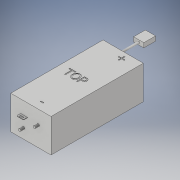
# Autodesk Inventor part: 12S Module
Saved by Autodesk Inventor 2017 (Build 210142000, 142)
## iProperties
Created: 2021-02-12
Part Number: 12S Module
Material: Generic
Document SubType Name: Modeling
Designer: Win240
Density: 1 g/cm^3
Appearance: Default
Author: Win240
Autodesk Inventor part; units mm, degrees
ref_plane "YZ Plane" through (0, 0, 0) normal (1, 0, 0) x (0, 1, 0)
ref_plane "XZ Plane" through (0, 0, 0) normal (0, 1, 0) x (-1, 0, 0)
ref_plane "XY Plane" through (0, 0, 0) normal (0, 0, 1) x (1, 0, 0)
sketch "Sketch1" plane through (0, 0, 0) normal (0, 0, 1) x (1, 0, 0)
  line L0 (-65.0875, -53.975) -> (65.0875, -53.975)
  line L1 (65.0875, -53.975) -> (65.0875, 53.975)
  line L2 (65.0875, 53.975) -> (-65.0875, 53.975)
  line L3 (-65.0875, 53.975) -> (-65.0875, -53.975)
  line L4 (-65.0875, -53.975) -> (65.0875, 53.975) construction
  line L5 (65.0875, -53.975) -> (-65.0875, 53.975) construction
  point P0 (0, 0)
  dimension "d0" = 130.175
  dimension "d1" = 107.95
  constraints: 12 end point, 2 midpoint, 2 parallel, 1 horizontal, 1 perpendicular
  measures "d0" distance of L0.start L0.end
  measures "d1" distance of L0.end L1.end
extrude "Extrusion1" add sketch "Sketch1" along normal blind 298.45
sketch "Sketch2" plane through (0, 0, 298.45) normal (0, 0, 1) x (1, 0, 0)
  line L0 (-65.0875, -53.975) -> (65.0875, -53.975) construction
  line L1 (-65.0875, 53.975) -> (-65.0875, -53.975) construction
  circle A0 centre (-23.8125, -22.225) radius 4
  circle A1 centre (23.8125, 9.525) radius 4
  line L2 (-11.1125, 12.065) -> (-33.3375, 12.065)
  line L3 (-33.3375, 12.065) -> (-33.3375, 13.335)
  line L4 (-33.3375, 13.335) -> (-11.1125, 13.335)
  line L5 (-11.1125, 13.335) -> (-11.1125, 12.065)
  line L6 (-33.3375, 12.7) -> (-65.0875, 12.7) construction
  point P0 (0, 0)
  dimension "d4" = 31.75
  dimension "d5" = 41.275
  dimension "d6" = 8
  dimension "d7" = 63.5
  dimension "d8" = 88.9
  dimension "d13" = 31.75
  dimension "d14" = 53.975
  dimension "d15" = 66.675
  dimension "d16" = 1.27
  constraints: 10 end point, 2 centre point, 2 horizontal, 2 parallel, 1 equal radius, 1 midpoint, 1 perpendicular, 1 point on line
  measures "d4" distance from line of A0.centre L0
  measures "d5" distance from line of A0.centre L1
  measures "d6" diameter of A0
  measures "d7" distance from line of A1.centre L0
  measures "d8" distance from line of A1.centre L1
  measures "d13" distance between parallel lines of L3 L1
  measures "d14" distance between parallel lines of L5 L1
  measures "d15" distance between parallel lines of L0 L6
  measures "d16" distance of L4.end L2.start
extrude "Extrusion2" add sketch "Sketch2" along normal blind 12.7
sketch "Sketch3" plane through (0, 0, 0) normal (0, 0, -1) x (-1, 0, 0)
  circle A0 centre (-23.8125, 9.525) radius 4 projected
  circle A1 centre (23.8125, -22.225) radius 4 projected
  line L0 (33.3375, 12.065) -> (11.1125, 12.065) projected
  line L1 (11.1125, 12.065) -> (11.1125, 13.335) projected
  line L2 (11.1125, 13.335) -> (33.3375, 13.335) projected
  line L3 (33.3375, 13.335) -> (33.3375, 12.065) projected
  point P0 (0, 0)
extrude "Extrusion3" add sketch "Sketch3" along normal blind 12.7
sketch "Sketch4" plane through (-33.3375, 13.335, 0) normal (0, 1, 0) x (1, 0, 0)
  line L0 (0, 12.7) -> (22.225, 12.7) projected
  line L1 (22.225, 0) -> (22.225, 12.7) projected
  line L2 (0, 0) -> (0, 12.7) projected
  line L3 (22.225, -298.45) -> (22.225, -311.15) projected
  line L4 (22.225, -311.15) -> (0, -311.15) projected
  line L5 (0, -298.45) -> (0, -311.15) projected
  line L6 (16.51, -308.61) -> (5.715, -308.61)
  line L7 (5.715, -308.61) -> (5.715, -304.165)
  line L8 (5.715, -304.165) -> (16.51, -304.165)
  line L9 (16.51, -304.165) -> (16.51, -308.61)
  line L10 (16.51, 5.715) -> (5.715, 5.715)
  line L11 (5.715, 5.715) -> (5.715, 10.16)
  line L12 (5.715, 10.16) -> (16.51, 10.16)
  line L13 (16.51, 10.16) -> (16.51, 5.715)
  line L14 (5.715, 10.16) -> (0, 12.7) construction
  line L15 (16.51, 10.16) -> (22.225, 12.7) construction
  line L16 (22.225, -311.15) -> (16.51, -308.61) construction
  line L17 (5.715, -308.61) -> (0, -311.15) construction
  point P0 (33.3375, 0)
  dimension "d17" = 10.795
  dimension "d18" = 6.985
  dimension "d19" = 2.54
  constraints: 24 end point, 5 equal length, 4 parallel, 2 horizontal, 2 perpendicular
  measures "d17" distance of L11.end L12.end
  measures "d18" distance between parallel lines of L10 L0
  measures "d19" distance between parallel lines of L12 L0
extrude "Extrusion4" cut sketch "Sketch4" against normal up to surface (1.27 mm away)
fillet "Fillet1" radius 3.175 4 edges at (-33.3375, 12.7, -12.7) (-11.1125, 12.7, -12.7) (-33.3375, 12.7, 311.15) (-11.1125, 12.7, 311.15)
thread "Thread1" size "M8x1.25" class "6g" standard "ANSI Metric M Profile" full length
thread "Thread2" size "M8x1.25" class "6g" standard "ANSI Metric M Profile" full length
thread "Thread3" size "M8x1.25" class "6g" standard "ANSI Metric M Profile" full length
thread "Thread4" size "M8x1.25" class "6g" standard "ANSI Metric M Profile" full length
sketch "Sketch5" plane through (-65.0875, 53.975, 0) normal (0, 1, 0) x (1, 0, 0)
  line L0 (25.2364, -11.8087) -> (114.825, -11.8087) construction
  line L1 (114.825, -11.8087) -> (114.825, -199.7093) construction
  line L2 (114.825, -199.7093) -> (25.2364, -199.7093) construction
  line L3 (25.2364, -199.7093) -> (25.2364, -11.8087) construction
  line L4 (91.6181, -23.1502) -> (83.0142, -23.1502)
  line L5 (83.0142, -23.1502) -> (83.0142, -31.7541)
  line L6 (83.0142, -31.7541) -> (80.1737, -31.7541)
  line L7 (80.1737, -31.7541) -> (80.1737, -23.1502)
  line L8 (80.1737, -23.1502) -> (71.5698, -23.1502)
  line L9 (71.5698, -23.1502) -> (71.5698, -20.4126)
  line L10 (71.5698, -20.4126) -> (80.1737, -20.4126)
  line L11 (80.1737, -20.4126) -> (80.1737, -11.8087)
  line L12 (80.1737, -11.8087) -> (83.0142, -11.8087)
  line L13 (83.0142, -11.8087) -> (83.0142, -20.4126)
  line L14 (83.0142, -20.4126) -> (91.6181, -20.4126)
  line L15 (91.6181, -20.4126) -> (91.6181, -23.1502)
  line L16 (33.7374, -158.3681) -> (33.7374, -135.9732)
  line L17 (33.7374, -135.9732) -> (25.2158, -135.9732)
  line L18 (25.2158, -135.9732) -> (25.2158, -132.9681)
  line L19 (25.2158, -132.9681) -> (45.6346, -132.9681)
  line L20 (45.6346, -132.9681) -> (45.6346, -135.9732)
  line L21 (45.6346, -135.9732) -> (37.1131, -135.9732)
  line L22 (37.1131, -135.9732) -> (37.1131, -158.3681)
  line L23 (37.1131, -158.3681) -> (33.7374, -158.3681)
  spline S0 degree 2 poles (66.1769, -135.8703) (67.6178, -137.5582) (69.2233, -142.4982) (69.2233, -145.6681) knots 0 0 0 1 2 2 2
  spline S1 degree 2 poles (69.2233, -145.6681) (69.2233, -148.7556) (67.6589, -153.7574) (66.1769, -155.4452) knots 0 0 0 1 2 2 2
  spline S2 degree 2 poles (66.1769, -155.4452) (64.6126, -157.2154) (60.4753, -158.9032) (57.9847, -158.9032) knots 0 0 0 1 2 2 2
  spline S3 degree 2 poles (57.9847, -158.9032) (55.4118, -158.9032) (51.2951, -157.1536) (49.7925, -155.4452) knots 0 0 0 1 2 2 2
  spline S4 degree 2 poles (49.7925, -155.4452) (48.3311, -153.7574) (46.7667, -148.7967) (46.7667, -145.6681) knots 0 0 0 1 2 2 2
  spline S5 degree 2 poles (46.7667, -145.6681) (46.7667, -142.4776) (48.3516, -137.6199) (49.8131, -135.8703) knots 0 0 0 1 2 2 2
  spline S6 degree 2 poles (49.8131, -135.8703) (51.2951, -134.1825) (55.4324, -132.4329) (57.9847, -132.4329) knots 0 0 0 1 2 2 2
  spline S7 degree 2 poles (57.9847, -132.4329) (60.5782, -132.4329) (64.7361, -134.2442) (66.1769, -135.8703) knots 0 0 0 1 2 2 2
  spline S8 degree 2 poles (65.7035, -145.6681) (65.7035, -143.1569) (64.6126, -139.2666) (63.6246, -137.9904) knots 0 0 0 1 2 2 2
  spline S9 degree 2 poles (63.6246, -137.9904) (62.616, -136.6731) (59.7755, -135.3557) (58.0053, -135.3557) knots 0 0 0 1 2 2 2
  spline S10 degree 2 poles (58.0053, -135.3557) (56.1734, -135.3557) (53.4152, -136.6319) (52.3654, -137.9904) knots 0 0 0 1 2 2 2
  spline S11 degree 2 poles (52.3654, -137.9904) (51.3568, -139.2872) (50.2865, -143.198) (50.2865, -145.6681) knots 0 0 0 1 2 2 2
  spline S12 degree 2 poles (50.2865, -145.6681) (50.2865, -150.6698) (54.4855, -155.9804) (58.0053, -155.9804) knots 0 0 0 1 2 2 2
  spline S13 degree 2 poles (58.0053, -155.9804) (61.5251, -155.9804) (65.7035, -150.6698) (65.7035, -145.6681) knots 0 0 0 1 2 2 2
  spline S14 degree 2 poles (88.9834, -140.6251) (88.9834, -142.2718) (87.8102, -145.2358) (86.7604, -146.265) knots 0 0 0 1 2 2 2
  spline S15 degree 2 poles (86.7604, -146.265) (85.4431, -147.5617) (81.8821, -148.8997) (79.1651, -148.8997) knots 0 0 0 1 2 2 2
  line L24 (79.1651, -148.8997) -> (76.304, -148.8997)
  line L25 (76.304, -148.8997) -> (76.304, -158.3681)
  line L26 (76.304, -158.3681) -> (72.9283, -158.3681)
  line L27 (72.9283, -158.3681) -> (72.9283, -132.9681)
  line L28 (72.9283, -132.9681) -> (79.3092, -132.9681)
  spline S16 degree 2 poles (79.3092, -132.9681) (81.5734, -132.9681) (84.7432, -133.7091) (85.9576, -134.553) knots 0 0 0 1 2 2 2
  spline S17 degree 2 poles (85.9576, -134.553) (87.3779, -135.5204) (88.9834, -138.505) (88.9834, -140.6251) knots 0 0 0 1 2 2 2
  spline S18 degree 2 poles (85.4636, -140.728) (85.4636, -139.4107) (84.558, -137.4758) (83.6317, -136.8583) knots 0 0 0 1 2 2 2
  spline S19 degree 2 poles (83.6317, -136.8583) (82.829, -136.3232) (80.6883, -135.8909) (79.1034, -135.8909) knots 0 0 0 1 2 2 2
  line L29 (79.1034, -135.8909) -> (76.304, -135.8909)
  line L30 (76.304, -135.8909) -> (76.304, -146.018)
  line L31 (76.304, -146.018) -> (78.6093, -146.018)
  spline S20 degree 2 poles (78.6093, -146.018) (80.6677, -146.018) (83.1995, -145.3593) (84.0228, -144.4948) knots 0 0 0 1 2 2 2
  spline S21 degree 2 poles (84.0228, -144.4948) (84.7844, -143.7332) (85.4636, -141.9424) (85.4636, -140.728) knots 0 0 0 1 2 2 2
  line L32 (80.0296, -274.258) -> (70.4171, -274.258)
  line L33 (70.4171, -274.258) -> (70.4171, -271.1705)
  line L34 (70.4171, -271.1705) -> (80.0296, -271.1705)
  line L35 (80.0296, -271.1705) -> (80.0296, -274.258)
  point P0 (65.0875, 0)
  constraints: 2 other
extrude "Extrusion7" cut sketch "Sketch5" against normal blind 0.762
sketch "Sketch6" plane through (0, 0, 0) normal (0, 0, -1) x (-1, 0, 0)
  circle A0 centre (8.3375, 46.3906) radius 3.175
  point P0 (0, 0)
  dimension "d31" = 6.35
  constraints: 1 centre point
  measures "d31" diameter of A0
extrude "Extrusion5" add sketch "Sketch6" along normal blind 58.42
sketch "Sketch7" plane through (-8.3375, 46.3906, -58.42) normal (0, 0, -1) x (-1, 0, 0)
  circle A0 centre (0, 0) radius 3.175 projected
  line L0 (-16.51, -7.3025) -> (16.51, -7.3025)
  line L1 (16.51, -7.3025) -> (16.51, 7.3025)
  line L2 (16.51, 7.3025) -> (-16.51, 7.3025)
  line L3 (-16.51, 7.3025) -> (-16.51, -7.3025)
  line L4 (-16.51, -7.3025) -> (16.51, 7.3025) construction
  line L5 (16.51, -7.3025) -> (-16.51, 7.3025) construction
  point P0 (-8.3375, -46.3906)
  dimension "d34" = 14.605
  dimension "d35" = 33.02
  constraints: 12 end point, 2 midpoint, 2 parallel, 1 horizontal, 1 perpendicular
  measures "d34" distance of L2.end L0.start
  measures "d35" distance of L1.end L2.end
extrude "Extrusion6" add sketch "Sketch7" along normal blind 38.1 contours A0 | L3 L2 L1 L0
body "Solid1"
